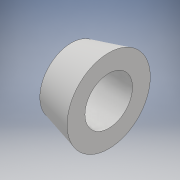
# Autodesk Inventor part: nutSecurer
Saved by Autodesk Inventor 2018 (Build 220112000, 112)
## iProperties
Created: 2017-10-29
Part Number: nutSecurer
Material: Generic
Document SubType Name: Modeling
Designer: Prakash
Density: 1 g/cm^3
Appearance: Default
Author: Prakash
Autodesk Inventor part; units mm, degrees
ref_plane "YZ Plane" through (0, 0, 0) normal (1, 0, 0) x (0, 1, 0)
ref_plane "XZ Plane" through (0, 0, 0) normal (0, 1, 0) x (-1, 0, 0)
ref_plane "XY Plane" through (0, 0, 0) normal (0, 0, 1) x (1, 0, 0)
sketch "Sketch1" plane through (0, 0, 0) normal (0, 1, 0) x (-1, 0, 0)
  line L0 (0, 0) -> (0, -11.1125)
  line L1 (5, -1.3562) -> (5, -9.7563)
  line L2 (0, 0) -> (5, -1.3562)
  line L3 (5, -9.7563) -> (0, -11.1125)
  line L4 (5, -5.5563) -> (0, -5.5563)
  dimension "d1" = 11.1125
  dimension "d2" = 8.4
  dimension "d3" = 5
  constraints: 10 end point, 2 midpoint, 2 vertical, 1 horizontal, 1 horizontal alignment
  measures "d1" distance of L0.start L0.end
  measures "d2" distance of L1.start L1.end
  measures "d3" distance between parallel lines of L0 L1
revolve "Revolution1" add sketch "Sketch1" angle 360 about axis through (-5, 0, -5.5563) along (1, 0, 0)
sketch "Sketch2" plane through (-5, 0, -5.5563) normal (-1, 0, 0) x (0, 0, 1)
  arc A0 (-4.2, 0) -> (4.2, 0) centre (0, 0) ccw projected
  circle A1 centre (0, 0) radius 3.175
  point P0 (5.5563, 0)
  dimension "d6" = 6.35
  constraints: 1 centre point, 1 coincident
  measures "d6" diameter of A1
extrude "Extrusion1" cut sketch "Sketch2" against normal up to surface (5 mm away)
body "Solid1"
